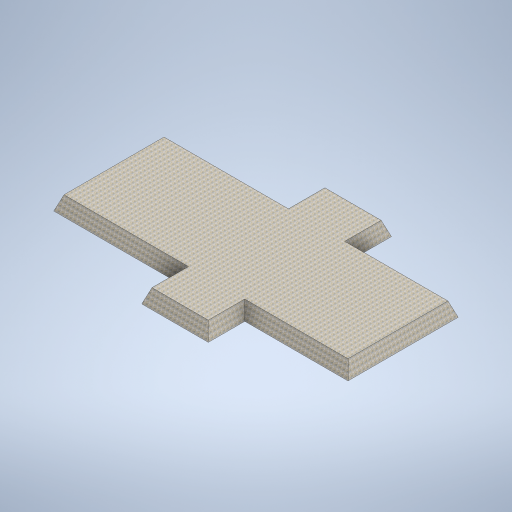
# Autodesk Inventor part: main_floor
Saved by Autodesk Inventor 2024.2 (Build 282272000, 272)
## iProperties
Created: 2024-05-24
Part Number: main_floor
Material: Limestone
Document SubType Name: Modeling
Designer: LOSTER_1
Density: 2.6 g/cm^3
Appearance: Limestone - Ashlar Coursed
Author: LOSTER_1
Autodesk Inventor part; units mm, degrees
ref_plane "YZ Plane" through (0, 0, 0) normal (1, 0, 0) x (0, 1, 0)
ref_plane "XZ Plane" through (0, 0, 0) normal (0, 1, 0) x (-1, 0, 0)
ref_plane "XY Plane" through (0, 0, 0) normal (0, 0, 1) x (1, 0, 0)
sketch "Sketch1" plane through (0, 0, 0) normal (0, 1, 0) x (-1, 0, 0)
  line L0 (-18589.1353, 7057.2083) -> (-18589.1353, -7090.0785)
  line L1 (18609.9901, -7090.0785) -> (18609.9901, 7057.2083)
  line L2 (18609.9901, 7057.2083) -> (21609.9901, 7057.2083)
  line L3 (21609.9901, 7057.2083) -> (21609.9901, -7090.0785)
  line L4 (21609.9901, -7090.0785) -> (18609.9901, -7090.0785)
  line L5 (18609.9901, -7090.0785) -> (18609.9901, 7057.2083)
  line L6 (-18589.1353, 7057.2083) -> (-21589.1353, 7057.2083)
  line L7 (-21589.1353, 7057.2083) -> (-21589.1353, -7090.0785)
  line L8 (-21589.1353, -7090.0785) -> (-18589.1353, -7090.0785)
  line L9 (-18589.1353, -7090.0785) -> (-18589.1353, 7057.2083)
  line L10 (18609.9901, 7057.2083) -> (3994.5778, 7057.2083)
  line L11 (-3973.723, 7057.2083) -> (-18589.1353, 7057.2083)
  line L12 (-18589.1353, -7090.0785) -> (-3973.723, -7090.0785)
  line L13 (3994.5778, -7090.0785) -> (18609.9901, -7090.0785)
  line L14 (3994.5778, -11251.4689) -> (3994.5778, -12251.4689)
  line L15 (3994.5778, -12251.4689) -> (1994.5778, -12251.4689)
  line L16 (-3973.723, 11218.7168) -> (-3973.723, 12218.7168)
  line L17 (-3973.723, 12218.7168) -> (-1973.723, 12218.7168)
  line L18 (3994.5778, -12251.4689) -> (-3973.723, -12251.4689)
  line L19 (-3973.723, -12251.4689) -> (-3973.723, 12218.7168)
  line L20 (-3973.723, 12218.7168) -> (3994.5778, 12218.7168)
  line L21 (3994.5778, 12218.7168) -> (3994.5778, -12251.4689)
  point P0 (1994.5778, 9218.7168)
  point P1 (1994.5778, -9251.4689)
  point P2 (-1973.723, -9251.4689)
  point P3 (-1973.723, -11251.4689)
  dimension "d0" = 3000
  dimension "d1" = 3000
  constraints: 44 end point, 11 parallel, 5 horizontal, 5 perpendicular, 5 point on line
  measures "d0" distance of L3.end L4.end
  measures "d1" distance of L8.end L7.end
extrude "Extrusion2" add sketch "Sketch1" against normal blind 2000 draft 20 contours L11 L19 L12 L0 | L19 L16 L17 L20 L21 L14 L15 L18 | L10 L1 L13 L21 | L2 L3 L4 L1
body "Solid2"
